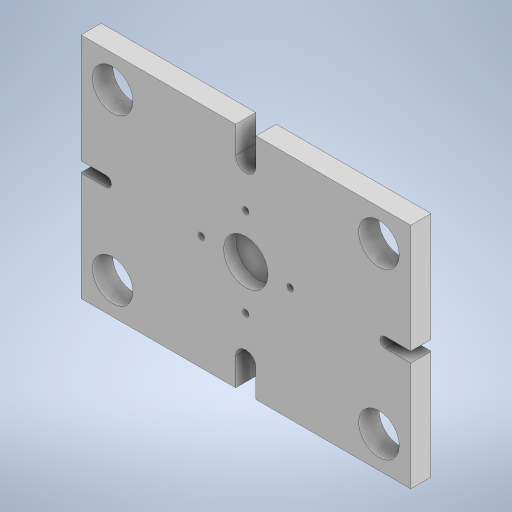
# Autodesk Inventor part: Base superior da ferramenta
Saved by Autodesk Inventor 2023.2 (Build 272271000, 271)
## iProperties
Created: 2022-04-25
Part Number: Base superior da ferramenta
Material: Generic
Document SubType Name: Modeling
Designer: coqui
Density: 1 g/cm^3
Appearance: Default
Mass: 672.993 g
Surface Area: 1109.82 cm^2
Volume: 672.993 cm^3
Author: coqui
Autodesk Inventor part; units mm, degrees
ref_plane "YZ Plane" through (0, 0, 0) normal (1, 0, 0) x (0, 1, 0)
ref_plane "XZ Plane" through (0, 0, 0) normal (0, 1, 0) x (-1, 0, 0)
ref_plane "XY Plane" through (0, 0, 0) normal (0, 0, 1) x (1, 0, 0)
sketch "Sketch1" plane through (0, 0, 0) normal (0, 0, 1) x (1, 0, 0)
  line L0 (130, 90) -> (-130, -90) construction
  line L1 (-130, 90) -> (130, -90) construction
  circle A0 centre (-105, 65) radius 16
  circle A1 centre (105, 65) radius 16
  circle A2 centre (105, -65) radius 16
  circle A3 centre (-105, -65) radius 16
  line L2 (0, -68.1117) -> (0, -128.2653) construction
  line L3 (-8, -68.1117) -> (-8, -90)
  line L4 (8, -90) -> (8, -68.1117)
  arc A4 (8, -68.1117) -> (-8, -68.1117) centre (0, -68.1117) ccw
  line L5 (138.2624, 0) -> (110, 0) construction
  line L6 (130, 4) -> (110, 4)
  line L7 (110, -4) -> (130, -4)
  arc A5 (110, 4) -> (110, -4) centre (110, 0) ccw
  line L8 (-67.4567, 0.3936) -> (51.9271, 0.3936) construction
  line L9 (0, -23.6129) -> (0, 33.7533) construction
  line L10 (-8, 68.899) -> (-8, 90)
  line L11 (8, 90) -> (8, 68.899)
  arc A6 (-8, 68.899) -> (8, 68.899) centre (0, 68.899) ccw
  line L12 (-130, -90) -> (-8, -90)
  line L13 (8, -90) -> (130, -90)
  line L14 (130, -90) -> (130, -4)
  line L15 (130, 4) -> (130, 90)
  line L16 (130, 90) -> (8, 90)
  line L17 (-8, 90) -> (-130, 90)
  line L18 (-130, 4) -> (-110, 4)
  line L19 (-110, -4) -> (-130, -4)
  arc A7 (-110, -4) -> (-110, 4) centre (-110, 0) ccw
  line L20 (-130, 90) -> (-130, 4)
  line L21 (-130, -4) -> (-130, -90)
  point P0 (0, 0)
  point P1 (4, -128.8323)
  point P2 (0, -98.1885)
  point P3 (124.1312, 0)
  point P4 (4, -87.7077)
  point P5 (130, 0)
  point P6 (-4, 128.8323)
  point P7 (4, 129.6196)
  dimension "d2" = 32
  dimension "d3" = 105
  dimension "d5" = 65
  dimension "d6" = 105
  dimension "d7" = 65
  dimension "d9" = 8
  dimension "d10" = 20
  dimension "d11" = 20
  dimension "d24" = 8
  dimension "d25" = 101
  dimension "d26" = 97
  dimension "d27" = 97
  dimension "d28" = 65
  dimension "d29" = 65
  dimension "d30" = 0
  dimension "d31" = 4
  dimension "d32" = 4
  dimension "d33" = 260
  dimension "d34" = 260
  dimension "d35" = 180
  dimension "d36" = 180
  constraints: 48 end point, 10 parallel, 9 symmetric about line, 8 centre point, 8 point on circle, 6 perpendicular, 4 midpoint, 4 tangent, 3 equal radius, 3 horizontal, 2 horizontal alignment, 2 vertical, 2 vertical alignment, 2 other
  measures "d2" diameter of A0
  measures "d3" horizontal distance of point (0, 0) A0.centre
  measures "d5" vertical distance of point (0, 0) A0.centre
  measures "d6" horizontal distance of point (0, 0) A1.centre
  measures "d7" vertical distance of point (0, 0) A2.centre
  measures "d9" diameter of A5
  measures "d10" distance of point (4, -87.708) L2.start
  measures "d11" distance of point (130, 0) L5.end
  measures "d24" radius of A4
  measures "d25" horizontal distance of A2.centre point (4, -87.708)
  measures "d26" horizontal distance of A2.centre L4.start
  measures "d27" horizontal distance of L3.end A3.centre
  measures "d28" vertical distance of L5.end A1.centre
  measures "d29" vertical distance of A7.centre A3.centre
  measures "d30" distance between parallel lines of L13 L12
  measures "d31" radius of A5
  measures "d32" radius of A7
  measures "d33" distance of L1.end L0.end
  measures "d34" distance of L0.start L1.start
  measures "d35" distance of L0.start L1.end
  measures "d36" distance of L1.start L0.end
extrude "Extrusion1" add sketch "Sketch1" along normal blind 16
sketch "Sketch2" plane through (0, 0, 16) normal (0, 0, 1) x (1, 0, 0)
  circle A0 centre (35, 0) radius 2.5
  point P0 (0, 0)
  dimension "d14" = 5
  dimension "d15" = 35
  constraints: 1 centre point
  measures "d14" diameter of A0
  measures "d15" distance of point (0, 0) A0.centre
extrude "Extrusion2" cut sketch "Sketch2" against normal blind 12
sketch "Sketch3" plane through (0, 0, 16) normal (0, 0, 1) x (1, 0, 0)
  circle A0 centre (0, 0) radius 17.5
  dimension "d18" = 35
  constraints: 1 centre point
  measures "d18" diameter of A0
extrude "Extrusion3" cut sketch "Sketch3" against normal blind 10
pattern_circular "Circular Pattern1" count 4 over 360 about axis through (0, 0, 16) along (0, 0, -1) of "Extrusion2"
body "Solid1"
